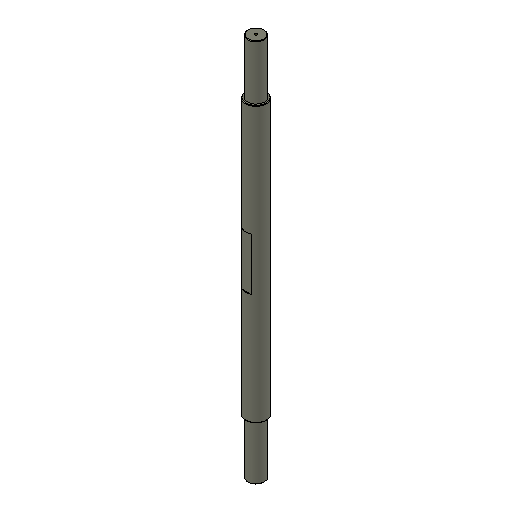
# Autodesk Inventor part: TL20240701-10120CV-008
Saved by Autodesk Inventor 2022.5 (Build 265521000, 521)
## iProperties
Category: FOLLOWER UNIT ASSY
Company: 현대 트랜시스(대유)
Created: 2023-01-26
Part Number: TL20240701-10120CV-008
Project: SW PJT
Checked By: 김형민
Engr Approved By: 김시현
User Status: 1 x18
Material: S45C
Description: 0
Document SubType Name: Modeling
Mfg Approved By: 호상태
Designer: 박성규
Stock Number: 008
Density: 7.87 g/cm^3
Appearance: Plating Kanizen
Mass: 6460.3 g
Surface Area: 896.596 cm^2
Volume: 820.877 cm^3
DETAIL: Coveryor Assembly
M/C TITLE: MEa/NEa차종 시트조립라인
SPECIFICATION: TL20221201-000000CV-034
Detail Description: Processed products
Title: SHAFT
Subject: SW차종 시트조립라인
Author: 박성규
Revision Number: A
Autodesk Inventor part; units mm, degrees
ref_plane "YZ Plane" through (0, 0, 0) normal (1, 0, 0) x (0, 1, 0)
ref_plane "XY Plane" through (0, 0, 0) normal (0, 0, 1) x (1, 0, 0)
sketch "스케치3" plane through (0, 0, 0) normal (0, 1, 0) x (-1, 0, 0)
  circle A0 centre (0, 0) radius 20
  dimension "d0" = 40
  constraints: 1 centre point, 1 coincident
  measures "d0" diameter of A0
extrude "돌출1" add sketch "스케치3" along normal mid plane 524
sketch "스케치4" plane through (0, -262, 0) normal (0, -1, 0) x (1, 0, 0)
  circle A0 centre (0, 0) radius 20 construction
  circle A1 centre (0, 0) radius 16
  dimension "d3" = 32
  constraints: 1 centre point, 1 coincident
  measures "d3" diameter of A1
extrude "돌출2" add sketch "스케치4" along normal blind 104
sketch "스케치5" plane through (0, 262, 0) normal (0, 1, 0) x (1, 0, 0)
  circle A0 centre (0, 0) radius 20 construction
  circle A1 centre (0, 0) radius 16
  dimension "d6" = 32
  constraints: 1 centre point, 1 coincident
  measures "d6" diameter of A1
extrude "돌출3" add sketch "스케치5" along normal blind 104
sketch "스케치6" plane through (0, 366, 0) normal (0, 1, 0) x (1, 0, 0)
  circle A0 centre (0, 0) radius 16 construction
  constraints: 1 coincident
hole "구멍1" at (0, 366, 0) direction (0, -1, 0) diameter 4.917 depth 17.1 tip angle 118 thread size "M6x1" class "6H" standard "ISO Metric profile"
sketch "스케치7" plane through (0, -366, 0) normal (0, -1, 0) x (1, 0, 0)
  circle A0 centre (0, 0) radius 16 construction
  constraints: 1 coincident
hole "구멍2" at (0, -366, 0) direction (0, 1, 0) diameter 4.917 depth 17.1 tip angle 118 thread size "M6x1" class "6H" standard "ISO Metric profile"
chamfer "모따기1" distance 1 angle 45 4 edges at (-16, -366, 0) (20, -262, 0) (20, 262, 0) (-16, 366, 0)
ref_plane "작업 평면1" through (0, 239.5, 0) normal (0, 1, 0) x (-1, 0, 0)
sketch "스케치9" plane through (0, 0, 0) normal (0, 1, 0) x (-1, 0, 0)
  circle A0 centre (0, 0) radius 20 projected
  line L0 (15, -25) -> (-15, -25)
  line L1 (-15, -25) -> (-15, -18)
  line L2 (-15, -18) -> (15, -18)
  line L3 (15, -18) -> (15, -25)
  line L4 (15, 18) -> (-15, 18)
  line L5 (-15, 18) -> (-15, 25)
  line L6 (-15, 25) -> (15, 25)
  line L7 (15, 25) -> (15, 18)
  point P0 (0, -25)
  point P1 (0, 18)
  point P2 (0, -18)
  point P3 (8.7178, -18)
  point P4 (-8.7178, -18)
  dimension "d36" = 18
  dimension "d37" = 7
  dimension "d38" = 30
  dimension "d39" = 18
  constraints: 16 end point, 4 parallel, 3 midpoint, 2 equal length, 2 horizontal, 2 perpendicular, 2 vertical alignment
  measures "d36" distance from line of point (0, 0) L2
  measures "d37" distance of L0.end L1.end
  measures "d38" distance of L0.start L0.end
  measures "d39" distance of point (0, 0) point (0, 18)
extrude "돌출5" cut sketch "스케치9" along normal mid plane 100 contours L4 A0 | A0 L4 L5 L6 L7 | L2 L3 L0 L1 A0 | A0 L2
